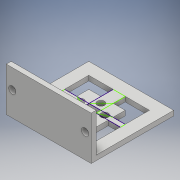
# Autodesk Inventor part: slide_sensor_base
Saved by Autodesk Inventor 2017 (Build 210142000, 142)
## iProperties
Created: 2019-03-03
Part Number: slide_sensor_base
Material: Generic
Document SubType Name: Modeling
Designer: simulator
Density: 1 g/cm^3
Appearance: Default
Author: simulator
## iProperties of the stored document slide_sensor_base_3DPrint.ipt
Created: 2019-03-05
Part Number: slide_sensor_base_3DPrint
Material: Generic
Document SubType Name: Modeling
Designer: simulator
Density: 1 g/cm^3
Appearance: Default
Author: simulator
Autodesk Inventor part; units mm, degrees
ref_plane "YZ Plane" through (0, 0, 0) normal (1, 0, 0) x (0, 1, 0)
ref_plane "XZ Plane" through (0, 0, 0) normal (0, 1, 0) x (-1, 0, 0)
ref_plane "XY Plane" through (0, 0, 0) normal (0, 0, 1) x (1, 0, 0)
sketch "Sketch1" plane through (0, 0, 0) normal (0, 1, 0) x (-1, 0, 0)
  line L0 (-30, 12) -> (-34, 12)
  line L1 (-34, 12) -> (-34, 14)
  line L2 (-34, 14) -> (-30, 14)
  line L3 (-30, 14) -> (-30, 16)
  line L4 (-30, 16) -> (-35, 16)
  line L5 (-35, 16) -> (-35, 0)
  line L6 (-35, 0) -> (-30, 0)
  line L7 (-30, 0) -> (-30, 12)
  line L8 (-1, 12) -> (-5, 12)
  line L9 (-5, 12) -> (-5, 0)
  line L10 (-5, 0) -> (0, 0)
  line L11 (0, 0) -> (0, 16)
  line L12 (0, 16) -> (-5, 16)
  line L13 (-5, 16) -> (-5, 14)
  line L14 (-5, 14) -> (-1, 14)
  line L15 (-1, 14) -> (-1, 12)
  line L16 (-35, 0) -> (0, 0)
  line L17 (0, 0) -> (0, -2)
  line L18 (0, -2) -> (-35, -2)
  line L19 (-35, -2) -> (-35, 0)
  line L20 (-35, 16) -> (0, 16)
  line L21 (0, 16) -> (0, -2)
  line L22 (0, -2) -> (-35, -2)
  line L23 (-35, -2) -> (-35, 16)
  line L24 (-35, 16) -> (-30, 0)
  line L25 (-5, 0) -> (0, 16)
  point P0 (-32.5, 8)
  point P1 (-2.5, 8)
  dimension "d0" = 2
  constraints: 52 end point, 4 parallel, 2 horizontal, 2 midpoint, 2 perpendicular
  measures "d0" distance of L16.end L17.end
extrude "Extrusion1" add sketch "Sketch1" along normal blind 32 contours L16 L10 L17 L18 L19 L6
extrude "Extrusion2" add sketch "Sketch1" against normal blind 2
hole "Hole1" at (32.5, 0, 8) at (2.5, 0, 8) direction (0, -1, 0) diameter 3 depth 8 tip angle 118
sketch "Sketch2" plane through (0, 32, 0) normal (0, 0, 1) x (1, 0, 0)
  line L0 (0, -32) -> (35, -32) projected
  line L1 (35, -32) -> (35, 0) projected
  line L2 (0, 0) -> (35, 0) projected
  line L3 (0, -32) -> (0, 0) projected
  line L4 (30, -5) -> (30, -27)
  line L5 (30, -27) -> (5, -27)
  line L6 (5, -27) -> (5, -5)
  line L7 (5, -5) -> (30, -5)
  line L8 (25, -22) -> (25, -10)
  line L9 (25, -10) -> (10, -10)
  line L10 (10, -10) -> (10, -22)
  line L11 (10, -22) -> (25, -22)
  line L12 (20, -15) -> (20, -17)
  line L13 (20, -17) -> (15, -17)
  line L14 (15, -17) -> (15, -15)
  line L15 (15, -15) -> (20, -15)
  point P0 (17.5, -5)
  point P1 (17.5, -10)
  point P2 (17.5, -27)
  point P3 (17.5, -22)
  point P4 (17.5, -15)
  point P5 (17.5, -17)
  dimension "d12" = 5
  dimension "d13" = 5
  dimension "d14" = 5
  constraints: 24 end point, 6 midpoint, 9 other
  measures "d12" distance between parallel lines of L1 L4
  measures "d13" distance between parallel lines of L4 L8
  measures "d14" distance between parallel lines of L8 L12
extrude "Extrusion3" cut sketch "Sketch2" against normal blind 10 contours L4 L5 L6 L7 | L12 L13 L14 L15
sketch "Sketch3" plane through (0, 32, 0) normal (0, 0, 1) x (1, 0, 0)
  line L0 (15, -17) -> (15, -15) projected
  line L1 (20, -15) -> (20, -17) projected
  line L2 (20, -17) -> (15, -17) projected
  line L3 (15, -15) -> (20, -15) projected
  line L4 (15, -17) -> (20, -17)
  line L5 (20, -17) -> (20, -28.4521)
  line L6 (20, -28.4521) -> (15, -28.4521)
  line L7 (15, -28.4521) -> (15, -17)
  line L8 (15, -15) -> (5, -15)
  line L9 (5, -15) -> (5, -17)
  line L10 (5, -17) -> (15, -17)
  line L11 (15, -17) -> (15, -15)
  line L12 (15, -15) -> (20, -15)
  line L13 (20, -15) -> (20, -5)
  line L14 (20, -5) -> (15, -5)
  line L15 (15, -5) -> (15, -15)
  line L16 (20, -15) -> (30, -15)
  line L17 (30, -15) -> (30, -17)
  line L18 (30, -17) -> (20, -17)
  line L19 (20, -17) -> (20, -15)
  line L20 (20, -10) -> (15, -15)
  line L21 (10, -15) -> (15, -17)
  line L22 (15, -17) -> (20, -22)
  line L23 (25, -15) -> (20, -17)
  point P0 (0, -32)
  point P1 (22.5, -16)
  point P2 (17.5, -12.5)
  point P3 (12.5, -16)
  point P4 (17.5, -19.5)
  constraints: 40 end point, 8 parallel, 7 midpoint, 5 perpendicular, 4 horizontal, 3 point on line
extrude "Extrusion4" add sketch "Sketch3" against normal up to surface (2 mm away) contours L22 L5 L6 L7 | L10 L9 L8 L21 | L2 L5 L22 | L15 L14 L13 L20 | L23 L16 L17 L18
hole "Hole2" at (22.5, 16, 0) at (17.5, 19.5, 0) at (12.5, 16, 0) at (17.5, 12.5, 0) direction (0, 0, -1) diameter 3 depth 8 tip angle 118
body "Solid1"
